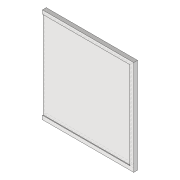
# Autodesk Inventor part: Ventil
Saved by Autodesk Inventor 2020 (Build 240168000, 168)
## iProperties
Created: 2020-04-08
Part Number: Ventil
Material: Generisch
Document SubType Name: Modeling
Designer: franz
Density: 1 g/cm^3
Appearance: Vorgabe
Author: franz
Autodesk Inventor part; units mm, degrees
ref_plane "YZ Plane" through (0, 0, 0) normal (1, 0, 0) x (0, 1, 0)
ref_plane "XZ Plane" through (0, 0, 0) normal (0, 1, 0) x (-1, 0, 0)
ref_plane "XY Plane" through (0, 0, 0) normal (0, 0, 1) x (1, 0, 0)
sketch "Skizze1" plane through (0, 0, 0) normal (0, 0, 1) x (1, 0, 0)
  line L0 (-115, -115) -> (115, -115)
  line L1 (115, -115) -> (115, 115)
  line L2 (115, 115) -> (-115, 115)
  line L3 (-115, 115) -> (-115, -115)
  line L4 (-115, -115) -> (115, 115) construction
  line L5 (115, -115) -> (-115, 115) construction
  point P0 (0, 0)
  dimension "d0" = 230
  dimension "d1" = 230
  constraints: 12 end point, 2 midpoint, 2 parallel, 1 horizontal, 1 perpendicular
  measures "d0" distance of L2.end L1.end
  measures "d1" distance of L1.end L0.end
extrude "Extrusion1" add sketch "Skizze1" along normal blind 3
sketch "Skizze2" plane through (0, 0, 0) normal (0, 0, -1) x (-1, 0, 0)
  line L0 (115, -125) -> (-125, -125)
  line L1 (-125, -125) -> (-125, 125)
  line L2 (-125, 125) -> (115, 125)
  line L3 (115, 125) -> (115, -125)
  line L4 (-115, 115) -> (115, 115) projected
  line L5 (-115, -115) -> (-115, 115) projected
  line L6 (115, -115) -> (-115, -115) projected
  point P0 (0, 0)
  dimension "d4" = 10
  dimension "d5" = 10
  dimension "d6" = 10
  constraints: 8 end point, 2 parallel, 1 horizontal, 1 perpendicular
  measures "d4" distance between parallel lines of L4 L2
  measures "d5" distance between parallel lines of L1 L5
  measures "d6" distance between parallel lines of L6 L0
extrude "Extrusion2" add sketch "Skizze2" against normal mid plane 10 contours L0 L1 L2 L3 L4 L5 L6
equation "\"d5\" = d4"
equation "\"d6\" = d4"
